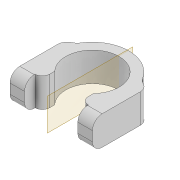
# Autodesk Inventor part: Arm_restriction_clip
Saved by Autodesk Inventor 2022 (Build 260153000, 153)
## iProperties
Created: 2022-07-25
Part Number: Arm_restriction_clip
Material: Generic
Document SubType Name: Modeling
Designer: dell
Density: 1 g/cm^3
Appearance: Default
Mass: 0.914716 g
Surface Area: 10.3779 cm^2
Volume: 0.914716 cm^3
Author: dell
Autodesk Inventor part; units mm, degrees
ref_plane "XZ Plane" through (0, 0, 0) normal (0, 1, 0) x (-1, 0, 0)
ref_plane "XY Plane" through (0, 0, 0) normal (0, 0, 1) x (1, 0, 0)
sketch "Sketch1" plane through (0, 0, 0) normal (0, 1, 0) x (-1, 0, 0)
  circle A0 centre (0, 0) radius 5.5
  circle A1 centre (0, 0) radius 7.5
  line L0 (7.5, 0) -> (-7.5, 0)
  line L1 (-7.5, 0) -> (-7.5, 8.5)
  line L2 (-7.5, 8.5) -> (7.5, 8.5)
  line L3 (7.5, 8.5) -> (7.5, 0)
  line L4 (5.5, 0) -> (-5.5, 0)
  line L5 (-5.5, 0) -> (-5.5, 8.5)
  line L6 (-5.5, 8.5) -> (5.5, 8.5)
  line L7 (5.5, 8.5) -> (5.5, 0)
  line L8 (4, 3.7749) -> (4, 6.3443)
  line L9 (-4, 3.7749) -> (-4, 6.3443)
  line L10 (4, 6.3443) -> (5.5, 6.3443)
  line L11 (-4, 6.3443) -> (-5.5, 6.3443)
  line L12 (-10.5, 0) -> (10.5, 0) projected
  point P0 (-5.5, 8.5)
  dimension "d0" = 11
  dimension "d1" = 2
  dimension "d3" = 1
  dimension "d4" = 1.5
  dimension "d5" = 1.5
  constraints: 24 end point, 8 point on circle, 6 point on line, 5 parallel, 3 perpendicular, 2 centre point, 1 coincident, 1 collinear, 1 horizontal, 1 vertical
  measures "d0" diameter of A0
  measures "d1" radial gap between concentric circles of A0 A1
  measures "d3" distance edge to line of A1 L2
  measures "d4" distance between parallel lines of L7 L8
  measures "d5" distance between parallel lines of L5 L9
extrude "Extrusion1" add sketch "Sketch1" along normal blind 6 contours L0 A1 A0 | L7 A1 L0 | A0 L8 A1 L7 | L5 A1 L9 A0 | L0 A1 L5 | A1 L7 L2 L3 | A1 L10 L7 | L1 L2 L5 A1 | L5 L11 A1
fillet "Fillet1" radius 1.5 2 edges at (-4, 3, 6.3443) (4, 3, 6.3443)
sketch "Sketch4" plane through (-7.5, 0, 0) normal (-1, 0, 0) x (0, 0, 1)
  line L0 (0, 0) -> (8.5, 0) projected
  line L1 (8.5, 0) -> (8.5, 6) projected
  line L2 (0, 6) -> (8.5, 6) projected
  line L3 (0, 0) -> (0, 6) projected
  line L4 (0, 0) -> (0, 0) projected
  line L5 (0, 0) -> (0, 6) projected
  line L6 (0, 6) -> (0, 6) projected
  line L7 (0, 0) -> (0, 6) projected
  line L8 (0, 0) -> (0, 6) projected
  line L9 (0, 6) -> (0, 0)
  line L10 (0, 0) -> (-3, 0)
  line L11 (-3, 0) -> (-3, 6)
  line L12 (-3, 6) -> (0, 6)
  point P0 (0, 0)
  dimension "d22" = 3
  constraints: 8 end point, 3 equal length, 1 perpendicular
  measures "d22" distance between parallel lines of L5 L11
extrude "Extrusion3" add sketch "Sketch4" along normal mid plane 2
fillet "Fillet2" radius 2 2 edges at (-8.5, 3, -3) (-6.8739, 3, -3)
mirror "Mirror1" about plane through (0, 0, 0) normal (1, 0, 0) of "Extrusion3", "Fillet2"
fillet "Fillet5" radius 2 4 edges at (7, 6, 8.5) (7, 0, 8.5) (-7, 6, 8.5) (-7, 0, 8.5)
body "Solid1"
